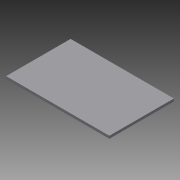
# Autodesk Inventor part: sensor_board_base
Saved by Autodesk Inventor 2013 (Build 170138000, 138)
## iProperties
Created: 2013-08-09
Part Number: sensor_board_base
Material: Generic
Document SubType Name: Modeling
Designer: Marc Bucchieri
Density: 1 g/cm^3
Author: Marc Bucchieri
Autodesk Inventor part; units mm, degrees
ref_plane "YZ Plane" through (0, 0, 0) normal (1, 0, 0) x (0, 1, 0)
ref_plane "XZ Plane" through (0, 0, 0) normal (0, 1, 0) x (-1, 0, 0)
ref_plane "XY Plane" through (0, 0, 0) normal (0, 0, 1) x (1, 0, 0)
sketch "Sketch1" plane through (0, 0, 0) normal (0, 1, 0) x (-1, 0, 0)
  line L0 (51.1438, -31.2785) -> (-50.4562, -31.2785)
  line L1 (-50.4562, -31.2785) -> (-50.4562, 32.2215)
  line L2 (-50.4562, 32.2215) -> (51.1438, 32.2215)
  line L3 (51.1438, 32.2215) -> (51.1438, -31.2785)
  line L4 (-67.5031, 0.4715) -> (104.603, 0.4715)
  point P0 (0, 0)
  dimension "d0" = 63.5
  dimension "d2" = 101.6
  dimension "d11" = 63.5
  constraints: 10 end point, 2 parallel, 2 perpendicular, 1 horizontal
  measures "d0" distance of L2.end L0.start
  measures "d2" distance of L0.start L0.end
  measures "d11" diameter of L0 L4
extrude "Extrusion1" add sketch "Sketch1" along normal blind 2.54
sketch "Sketch2" plane through (0, 0, 0) normal (0, -1, 0) x (1, 0, 0)
  line L0 (-51.1438, -31.2785) -> (50.4562, -31.2785) projected
  line L1 (50.4562, -31.2785) -> (50.4562, 32.2215) projected
  line L2 (50.4562, 32.2215) -> (-51.1438, 32.2215) projected
  line L3 (-51.1438, 32.2215) -> (-51.1438, -31.2785) projected
  circle A0 centre (-40.9838, 0) radius 3.175
  circle A1 centre (40.2962, 22.0615) radius 3.175
  circle A2 centre (40.2962, -21.1185) radius 3.175
  line L4 (40.2962, 22.0615) -> (40.2962, -21.1185) construction
  point P0 (0, 0)
  dimension "d5" = 6.35
  dimension "d6" = 10.16
  dimension "d7" = 6.35
  dimension "d8" = 10.16
  dimension "d9" = 10.16
  dimension "d12" = 6.35
  dimension "d13" = 10.16
  constraints: 3 centre point, 2 coincident, 2 end point, 1 vertical
  measures "d5" diameter of A0
  measures "d6" distance from line of L3 A0.centre
  measures "d7" diameter of A1
  measures "d8" distance from line of L1 A1.centre
  measures "d9" distance from line of L2 A1.centre
  measures "d12" diameter of A2
  measures "d13" distance from line of L0 L4.end
extrude "Extrusion2" add sketch "Sketch2" along normal blind 2.032 contours A0 | A1 | A2
body "Solid1"
